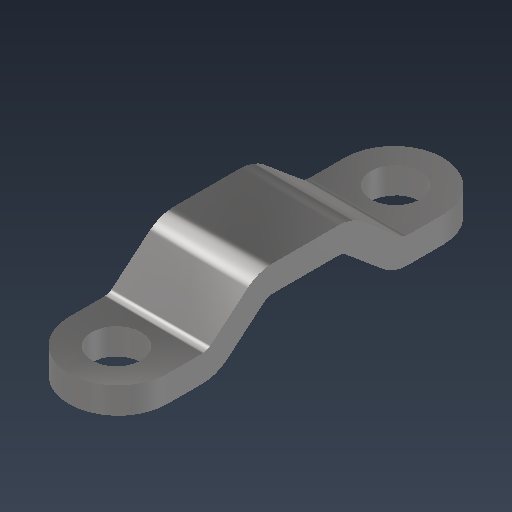
# Autodesk Inventor part: SP7V1 Viela Freno
Saved by Autodesk Inventor 2021.2 (Build 252289000, 289)
## iProperties
Created: 2026-07-29
Part Number: SP7V1 Viela Freno
Material: Stainless Steel
Document SubType Name: Sheet Metal
Designer: Tecnica
Density: 8.08 g/cm^3
Sheet Metal Rule: Default_mm
Appearance: Semi-Polished
Flat Pattern Width: 1.2 cm
Flat Pattern Length: 4.66139 cm
Flat Pattern Area: 5.59367 cm^2
Sheet Metal Width: 12.000 mm
Sheet Metal Length: 46.614 mm
Sheet Metal Area: 559.367 mm^2
Mass: 12.9532 g
Surface Area: 14.8025 cm^2
Volume: 1.60312 cm^3
Author: Tecnica
Autodesk Inventor part; units mm, degrees
ref_plane "YZ Plane" through (0, 0, 0) normal (1, 0, 0) x (0, 1, 0)
ref_plane "XZ Plane" through (0, 0, 0) normal (0, 1, 0) x (-1, 0, 0)
ref_plane "XY Plane" through (0, 0, 0) normal (0, 0, 1) x (1, 0, 0)
sketch "Sketch1" plane through (0, 0, 0) normal (0, 1, 0) x (-1, 0, 0)
  line L0 (-6, 4) -> (6, 4)
  line L1 (6, 4) -> (6, -4)
  line L2 (6, -4) -> (-6, -4)
  line L3 (-6, -4) -> (-6, 4)
  line L4 (-6, 4) -> (6, -4) construction
  line L5 (6, 4) -> (-6, -4) construction
  point P0 (0, 0)
  dimension "d0" = 12
  dimension "d1" = 8
  measures "d0" distance of L1.end L2.end
  measures "d1" distance of L0.end L1.end
extrude "Plate1" add sketch "Sketch1" along normal blind 3.2
sketch "Sketch2" plane through (-6, -0.3547, -4.9745) normal (0, 0.7660444, -0.6427876) x (1, 0, 0)
  line L0 (12, 0) -> (0, 0)
  line L1 (0, 0) -> (0, -5.8835)
  line L2 (0, -5.8835) -> (12, -5.8835)
  line L3 (12, -5.8835) -> (12, 0)
  constraints: 6 end point, 1 horizontal, 1 perpendicular, 1 vertical
edge flange "Flange1" height 7.6 angle 40 thickness 3.2 bend radius 1.516 thickness toward (0, 0.7660444, -0.6427876) relief tear relief width 3.2 relief depth 1.6 edges at (0, 3.2, -4) wall of the first edge with corners at (6, -0.3547, -4.9745) (-6, -0.3547, -4.9745) (-6, -4.1365, -9.4815) (6, -4.1365, -9.4815)
bend "Bend1"
corner "Corner1"
sketch "Sketch3" plane through (6, -2.0399, -12.5129) normal (0, -1, 0) x (-1, 0, 0)
  line L0 (12, 0) -> (0, 0)
  line L1 (0, 0) -> (0, -10.2835)
  line L2 (0, -10.2835) -> (12, -10.2835)
  line L3 (12, -10.2835) -> (12, 0)
  constraints: 6 end point, 1 horizontal, 1 perpendicular, 1 vertical
edge flange "Flange2" height 12 angle 40 thickness 3.2 bend radius 1.516 thickness toward (0, -1, 0) relief tear relief width 3.2 relief depth 1.6 edges at (0, -4.1365, -9.4815) wall of the first edge with corners at (-6, -2.0399, -12.5129) (6, -2.0399, -12.5129) (6, -2.0399, -22.7964) (-6, -2.0399, -22.7964)
bend "Bend2"
corner "Corner2"
sketch "Sketch4" plane through (6, -0.3547, 4.9745) normal (0, 0.7660444, 0.6427876) x (1, 0, 0)
  line L0 (-12, 0) -> (0, 0)
  line L1 (0, 0) -> (0, 5.8835)
  line L2 (0, 5.8835) -> (-12, 5.8835)
  line L3 (-12, 5.8835) -> (-12, 0)
  constraints: 6 end point, 1 horizontal, 1 perpendicular, 1 vertical
edge flange "Flange3" height 7.6 angle 40 thickness 3.2 bend radius 1.516 thickness toward (0, 0.7660444, 0.6427876) relief tear relief width 3.2 relief depth 1.6 edges at (0, 3.2, 4) wall of the first edge with corners at (-6, -0.3547, 4.9745) (6, -0.3547, 4.9745) (6, -4.1365, 9.4815) (-6, -4.1365, 9.4815)
bend "Bend3"
corner "Corner3"
sketch "Sketch5" plane through (-6, -2.0399, 12.5129) normal (0, -1, 0) x (-1, 0, 0)
  line L0 (-12, 0) -> (0, 0)
  line L1 (0, 0) -> (0, 10.2835)
  line L2 (0, 10.2835) -> (-12, 10.2835)
  line L3 (-12, 10.2835) -> (-12, 0)
  constraints: 6 end point, 1 horizontal, 1 perpendicular, 1 vertical
edge flange "Flange4" height 12 angle 40 thickness 3.2 bend radius 1.516 thickness toward (0, -1, 0) relief tear relief width 3.2 relief depth 1.6 edges at (0, -4.1365, 9.4815) wall of the first edge with corners at (6, -2.0399, 12.5129) (-6, -2.0399, 12.5129) (-6, -2.0399, 22.7964) (6, -2.0399, 22.7964)
bend "Bend4"
corner "Corner4"
fillet "Fillet1" radius 6 4 edges at (6, -3.6399, -22.7964) (-6, -3.6399, -22.7964) (6, -3.6399, 22.7964) (-6, -3.6399, 22.7964)
sketch "Sketch6" plane through (-6, -2.0399, 12.5129) normal (0, 1, 0) x (1, 0, 0)
  arc A0 (0, -4.2835) -> (12, -4.2835) centre (6, -4.2835) ccw projected
  line L0 (6, -10.2835) -> (6, 35.3093)
  arc A1 (12, 29.3093) -> (0, 29.3093) centre (6, 29.3093) ccw projected
  line L1 (6, 12.5129) -> (6, -4.4871)
  circle A2 centre (6, -4.4871) radius 3
  line L2 (6, 12.5129) -> (6, 29.5129)
  circle A3 centre (6, 29.5129) radius 3
  dimension "d50" = 17
  dimension "d51" = 6
  dimension "d52" = 17
  dimension "d53" = 6
  constraints: 6 end point, 2 centre point, 2 coincident, 2 point on circle, 2 point on line, 1 vertical
  measures "d50" distance of L1.start L1.end
  measures "d51" diameter of A2
  measures "d52" distance of L1.start L2.end
  measures "d53" diameter of A3
extrude "Cut1" cut sketch "Sketch6" against normal blind 3.2
equation "\"d54\" = Thickness"
equation "\"d2\" = Thickness"
equation "\"d3\" = BendReliefWidth"
equation "\"d4\" = BendReliefDepth"
equation "\"d5\" = MinimumRemnant"
equation "\"d6\" = TransitionRadius"
equation "\"d9\" = BendRadius"
equation "\"d10\" = CornerReliefSize"
equation "\"d11\" = GapSize"
equation "\"d12\" = JacobiRadiusSize"
equation "\"d13\" = BendReliefWidth"
equation "\"d14\" = BendReliefDepth"
equation "\"d15\" = MinimumRemnant"
equation "\"d16\" = TransitionRadius"
equation "\"d19\" = BendRadius"
equation "\"d20\" = CornerReliefSize"
equation "\"d21\" = GapSize"
equation "\"d22\" = JacobiRadiusSize"
equation "\"d23\" = BendReliefWidth"
equation "\"d24\" = BendReliefDepth"
equation "\"d25\" = MinimumRemnant"
equation "\"d26\" = TransitionRadius"
equation "\"d29\" = BendRadius"
equation "\"d30\" = CornerReliefSize"
equation "\"d31\" = GapSize"
equation "\"d32\" = JacobiRadiusSize"
equation "\"d33\" = BendReliefWidth"
equation "\"d34\" = BendReliefDepth"
equation "\"d35\" = MinimumRemnant"
equation "\"d36\" = TransitionRadius"
equation "\"d39\" = BendRadius"
equation "\"d40\" = CornerReliefSize"
equation "\"d41\" = GapSize"
equation "\"d42\" = JacobiRadiusSize"
equation "\"BendReliefWidth\" = Thickness"
equation "\"BendReliefDepth\" = 0.5 * Thickness"
equation "\"CornerReliefSize\" = 4 * Thickness"
equation "\"MinimumRemnant\" = 2 * Thickness"
equation "\"TransitionRadius\" = BendRadius"
equation "\"JacobiRadiusSize\" = BendRadius"
equation "\"GapSize\" = Thickness"
equation "\"Thickness\" = 3.2"
equation "\"BendRadius\" = 1.516"
body "Solid1"
